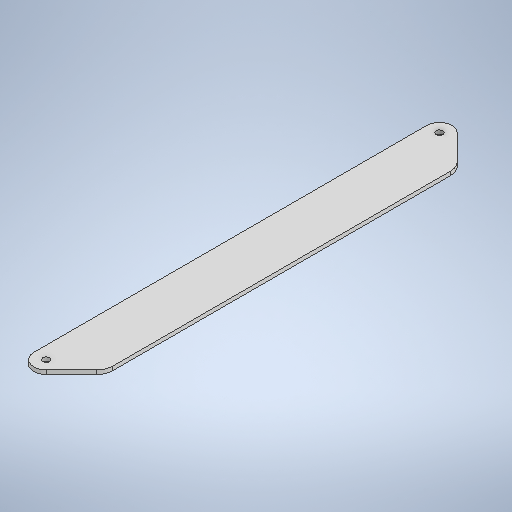
# Autodesk Inventor part: A3P2
Saved by Autodesk Inventor 2025.2 (Build 292293000, 293)
## iProperties
Created: 2025-05-22
Part Number: A3P2
Material: Generic
Document SubType Name: Sheet Metal
Designer: Admin
Density: 1 g/cm^3
Sheet Metal Rule: Default
Appearance: Default
Author: Admin
Autodesk Inventor part; units mm, degrees
ref_plane "YZ Plane" through (0, 0, 0) normal (1, 0, 0) x (0, 1, 0)
ref_plane "XZ Plane" through (0, 0, 0) normal (0, 1, 0) x (-1, 0, 0)
ref_plane "XY Plane" through (0, 0, 0) normal (0, 0, 1) x (1, 0, 0)
sketch "Sketch1" plane through (0, 0, 0) normal (0, 1, 0) x (-1, 0, 0)
  arc A0 (5.45, 0) -> (-3.8537, 3.8537) centre (0, 0) ccw
  line L0 (5.45, 0) -> (5.45, -170)
  line L1 (-3.8537, 3.8537) -> (-14.7075, -7)
  arc A1 (-14.7075, -7) -> (-16.7785, -12) centre (-9.7075, -12) ccw
  line L2 (-16.7785, -12) -> (-16.7785, -158)
  arc A2 (-3.8537, -173.8537) -> (5.45, -170) centre (0, -170) ccw
  line L3 (-3.8537, -173.8537) -> (-14.7075, -163)
  arc A3 (-16.7785, -158) -> (-14.7075, -163) centre (-9.7075, -158) ccw
  dimension "d0" = 10.9
  dimension "d3" = 170
  dimension "d5" = 0
  dimension "d6" = 12
  dimension "d7" = 12
  dimension "d8" = 5.45
  dimension "d9" = 45
  dimension "d10" = 7
  dimension "d11" = 7
  dimension "d12" = 10.9
  dimension "d13" = 135
  constraints: 8 end point, 8 point on circle, 5 tangent, 4 centre point, 2 vertical, 1 coincident
  measures "d0" diameter of A0
  measures "d3" distance of A2.centre point (0, 0)
  measures "d5" horizontal distance of A2.centre point (0, 0)
  measures "d6" vertical distance of L2.start point (0, 0)
  measures "d7" vertical distance of L2.end A2.centre
  measures "d8" distance from line of point (0, 0) L0
  measures "d9" angle of L0 L1
  measures "d10" vertical distance of point (0, 0) L1.end
  measures "d11" vertical distance of A2.centre L3.end
  measures "d12" diameter of A2
  measures "d13" angle of L3 L0
extrude "Extrusion1" add sketch "Sketch1" along normal blind 1.7
sketch "Sketch2" plane through (0, 1.7, 0) normal (0, 1, 0) x (1, 0, 0)
  arc A0 (3.8537, 173.8537) -> (-5.45, 170) centre (0, 170) ccw projected
  arc A1 (-5.45, 0) -> (3.8537, -3.8537) centre (0, 0) ccw projected
  circle A2 centre (0, 0) radius 1.5
  circle A3 centre (0, 170) radius 1.5
  dimension "d16" = 3
  dimension "d17" = 3
  constraints: 2 centre point, 2 coincident
  measures "d16" diameter of A2
  measures "d17" diameter of A3
extrude "Extrusion2" cut sketch "Sketch2" against normal blind 1.7
equation "\"BendRadius\" = Thickness"
equation "\"BendReliefWidth\" = Thickness"
equation "\"BendReliefDepth\" = 0.5 * Thickness"
equation "\"CornerReliefSize\" = 4 * Thickness"
equation "\"MinimumRemnant\" = 2 * Thickness"
equation "\"TransitionRadius\" = BendRadius"
equation "\"JacobiRadiusSize\" = BendRadius"
equation "\"GapSize\" = Thickness"
equation "\"Thickness\" = 3.048"
body "Solid1"
